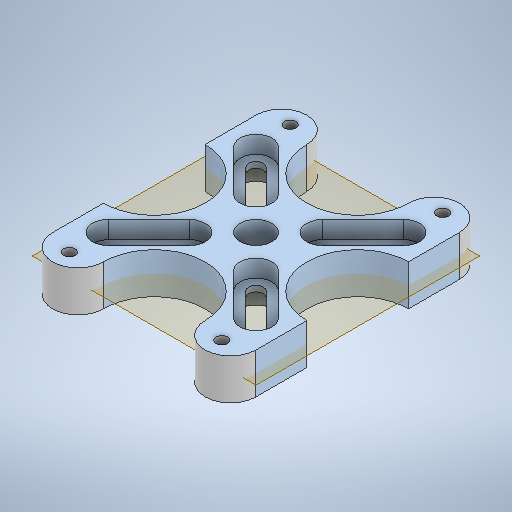
# Autodesk Inventor part: BaseSketchGrabberrev2.0
Saved by Autodesk Inventor 2025.1 (Build 291241000, 241)
## iProperties
Created: 2024-09-22
Part Number: BaseSketchGrabberrev2.0
Material: Generic
Document SubType Name: Modeling
Designer: m_kni
Density: 1 g/cm^3
Appearance: Default
Author: m_kni
Autodesk Inventor part; units mm, degrees
ref_plane "YZ Plane" through (0, 0, 0) normal (1, 0, 0) x (0, 1, 0)
ref_plane "XZ Plane" through (0, 0, 0) normal (0, 1, 0) x (-1, 0, 0)
ref_plane "XY Plane" through (0, 0, 0) normal (0, 0, 1) x (1, 0, 0)
sketch "Sketch1" plane through (0, 0, 0) normal (0, 1, 0) x (-1, 0, 0)
  line L0 (-12.7, 12.7) -> (12.7, 12.7)
  line L1 (12.7, 12.7) -> (12.7, -12.7)
  line L2 (12.7, -12.7) -> (-12.7, -12.7)
  line L3 (-12.7, -12.7) -> (-12.7, 12.7)
  line L4 (-12.7, 12.7) -> (12.7, -12.7) construction
  line L5 (12.7, 12.7) -> (-12.7, -12.7) construction
  line L6 (-11.4786, 11.4786) -> (11.4786, 11.4786)
  line L7 (11.4786, 11.4786) -> (11.4786, -11.4786)
  line L8 (11.4786, -11.4786) -> (-11.4786, -11.4786)
  line L9 (-11.4786, -11.4786) -> (-11.4786, 11.4786)
  line L10 (-11.4786, 11.4786) -> (11.4786, -11.4786) construction
  line L11 (11.4786, 11.4786) -> (-11.4786, -11.4786) construction
  line L12 (-25.4, -25.4) -> (25.4, -25.4)
  line L13 (25.4, -25.4) -> (25.4, 25.4)
  line L14 (25.4, 25.4) -> (-25.4, 25.4)
  line L15 (-25.4, 25.4) -> (-25.4, -25.4)
  line L16 (-25.4, -25.4) -> (25.4, 25.4) construction
  line L17 (25.4, -25.4) -> (-25.4, 25.4) construction
  circle A0 centre (0, 0) radius 5.5
  circle A1 centre (11.4786, 11.4786) radius 5.5
  circle A2 centre (11.4786, -11.4786) radius 5.5
  circle A3 centre (-11.4786, 11.4786) radius 5.5
  circle A4 centre (-11.4786, -11.4786) radius 5.5
  circle A5 centre (-25.4, 25.4) radius 5.5
  circle A6 centre (25.4, 25.4) radius 5.5
  circle A7 centre (25.4, -25.4) radius 5.5
  circle A8 centre (-25.4, -25.4) radius 5.5
  line L18 (7.5895, 15.3677) -> (21.5109, 29.2891)
  line L19 (29.2891, 21.5109) -> (15.3677, 7.5895)
  line L20 (15.3677, -7.5895) -> (29.2891, -21.5109)
  line L21 (-7.5895, -15.3677) -> (-21.5109, -29.2891)
  line L22 (-29.2891, 21.5109) -> (-15.3677, 7.5895)
  line L23 (7.5895, -15.3677) -> (21.5109, -29.2891)
  line L24 (-15.3677, -7.5895) -> (-29.2891, -21.5109)
  line L25 (-7.5895, 15.3677) -> (-21.5109, 29.2891)
  line L26 (-35, -35) -> (35, -35)
  line L27 (35, -35) -> (35, 35)
  line L28 (35, 35) -> (-35, 35)
  line L29 (-35, 35) -> (-35, -35)
  line L30 (-35, -35) -> (35, 35) construction
  line L31 (35, -35) -> (-35, 35) construction
  circle A9 centre (11.4786, 11.4786) radius 2.5
  circle A10 centre (25.4, 25.4) radius 2.5
  line L32 (27.1678, 23.6322) -> (13.2464, 9.7109)
  line L33 (23.6322, 27.1678) -> (9.7109, 13.2464)
  line L34 (0, 0) -> (0, 35)
  line L35 (35, 0) -> (0, 0)
  circle A11 centre (-11.4786, 11.4786) radius 2.5
  circle A12 centre (-25.4, 25.4) radius 2.5
  line L36 (-27.1678, 23.6322) -> (-13.2464, 9.7109)
  line L37 (-23.6322, 27.1678) -> (-9.7109, 13.2464)
  line L38 (25.4, 25.4) -> (-25.4, -25.4) construction
  circle A13 centre (11.4786, -11.4786) radius 2.5
  circle A14 centre (25.4, -25.4) radius 2.5
  line L39 (27.1678, -23.6322) -> (13.2464, -9.7109)
  line L40 (23.6322, -27.1678) -> (9.7109, -13.2464)
  line L41 (-27.1678, -23.6322) -> (-13.2464, -9.7109)
  circle A15 centre (-25.4, -25.4) radius 2.5
  line L42 (-23.6322, -27.1678) -> (-9.7109, -13.2464)
  circle A16 centre (-11.4786, -11.4786) radius 2.5
  dimension "d0" = 25.4
  dimension "d1" = 25.4
  dimension "d4" = 50.8
  dimension "d5" = 50.8
  dimension "d6" = 11
  dimension "d7" = 11
  dimension "d8" = 11
  dimension "d9" = 11
  dimension "d10" = 11
  dimension "d11" = 11
  dimension "d12" = 11
  dimension "d13" = 11
  dimension "d14" = 11
  dimension "d15" = 70
  dimension "d16" = 5
  dimension "d17" = 5
  constraints: 86 end point, 32 point on circle, 18 symmetric about line, 17 centre point, 13 tangent, 11 coincident, 10 midpoint, 8 parallel, 5 horizontal, 5 perpendicular, 3 point on line, 6 other
  measures "d0" distance of L1.end L2.end
  measures "d1" distance of L0.end L1.end
  measures "d4" distance of L14.end L13.end
  measures "d5" distance of L13.end L12.end
  measures "d6" diameter of A0
  measures "d7" diameter of A1
  measures "d8" diameter of A2
  measures "d9" diameter of A3
  measures "d10" diameter of A4
  measures "d11" diameter of A5
  measures "d12" diameter of A6
  measures "d13" diameter of A7
  measures "d14" diameter of A8
  measures "d15" distance of L28.end L27.end
  measures "d16" diameter of A9
  measures "d17" diameter of A10
extrude "Extrusion1" add sketch "Sketch1" along normal blind 14 contours A3 L25 L14 L34 L0 | L0 L34 L6 A3 | A3 L9 A4 L3 | L3 A4 L24 L15 L22 A3 | L34 L14 L18 A1 L0 | L0 A1 L6 L34 | L6 L34 A0 L35 L7 A2 L8 A4 L9 A3 | L6 A1 L7 L35 A0 L34 | L34 L28 L27 L35 L13 L19 A6 L18 L14 | L14 L25 A5 L22 L15 L24 A8 L21 L12 L23 A7 L20 L13 L35 L27 L26 L29 L28 L34 | L8 A2 L2 A4 | A1 L1 L35 L7 | L2 A2 L23 L12 L21 A4 | L35 L1 A2 L7 | A1 L19 L13 L35 L1 | L35 L13 L20 A2 L1
ref_plane "Work Plane1" through (0, 7, 0) normal (0, 1, 0) x (1, 0, 0)
sketch "Sketch3" plane through (0, 7, 0) normal (0, 1, 0) x (1, 0, 0)
  line L0 (-12.7, 12.7) -> (12.7, 12.7)
  line L1 (12.7, 12.7) -> (12.7, -12.7)
  line L2 (12.7, -12.7) -> (-12.7, -12.7)
  line L3 (-12.7, -12.7) -> (-12.7, 12.7)
  line L4 (-12.7, 12.7) -> (12.7, -12.7) construction
  line L5 (12.7, 12.7) -> (-12.7, -12.7) construction
  line L6 (-11.4786, 11.4786) -> (11.4786, 11.4786)
  line L7 (11.4786, 11.4786) -> (11.4786, -11.4786)
  line L8 (11.4786, -11.4786) -> (-11.4786, -11.4786)
  line L9 (-11.4786, -11.4786) -> (-11.4786, 11.4786)
  line L10 (-11.4786, 11.4786) -> (11.4786, -11.4786) construction
  line L11 (11.4786, 11.4786) -> (-11.4786, -11.4786) construction
  line L12 (-25.4, -25.4) -> (25.4, -25.4)
  line L13 (25.4, -25.4) -> (25.4, 25.4)
  line L14 (25.4, 25.4) -> (-25.4, 25.4)
  line L15 (-25.4, 25.4) -> (-25.4, -25.4)
  line L16 (-25.4, -25.4) -> (25.4, 25.4) construction
  line L17 (25.4, -25.4) -> (-25.4, 25.4) construction
  circle A0 centre (0, 0) radius 5.5
  circle A1 centre (11.4786, 11.4786) radius 5.5
  circle A2 centre (11.4786, -11.4786) radius 5.5
  circle A3 centre (-11.4786, 11.4786) radius 5.5
  circle A4 centre (-11.4786, -11.4786) radius 5.5
  circle A5 centre (-25.4, 25.4) radius 5.5
  circle A6 centre (25.4, 25.4) radius 5.5
  circle A7 centre (25.4, -25.4) radius 5.5
  circle A8 centre (-25.4, -25.4) radius 5.5
  line L18 (7.5895, 15.3677) -> (21.5109, 29.2891)
  line L19 (29.2891, 21.5109) -> (15.3677, 7.5895)
  line L20 (15.3677, -7.5895) -> (29.2891, -21.5109)
  line L21 (-7.5895, -15.3677) -> (-21.5109, -29.2891)
  line L22 (-29.2891, 21.5109) -> (-15.3677, 7.5895)
  line L23 (7.5895, -15.3677) -> (21.5109, -29.2891)
  line L24 (-15.719, -7.9759) -> (-29.6403, -21.8972)
  line L25 (-7.5895, 15.3677) -> (-21.5109, 29.2891)
  line L26 (-35, -35) -> (35, -35)
  line L27 (35, -35) -> (35, 35)
  line L28 (35, 35) -> (-35, 35)
  line L29 (-35, 35) -> (-35, -35)
  line L30 (-35, -35) -> (35, 35) construction
  line L31 (35, -35) -> (-35, 35) construction
  circle A9 centre (11.4786, 11.4786) radius 2.5
  circle A10 centre (25.4, 25.4) radius 2.5
  line L32 (27.1678, 23.6322) -> (13.2464, 9.7109)
  line L33 (23.58, 27.1139) -> (9.711, 13.2465)
  line L34 (0, 0) -> (0, 35)
  line L35 (35, 0) -> (0, 0)
  line L36 (-27.1678, 23.6322) -> (-13.2464, 9.7109)
  circle A11 centre (-25.4, 25.4) radius 2.5
  line L37 (-23.58, 27.1139) -> (-9.711, 13.2465)
  circle A12 centre (-11.4786, 11.4786) radius 2.5
  circle A13 centre (25.4, -25.4) radius 2.5
  line L38 (23.58, -27.1139) -> (9.711, -13.2465)
  line L39 (27.1678, -23.6322) -> (13.2464, -9.7109)
  circle A14 centre (11.4786, -11.4786) radius 2.5
  circle A15 centre (-11.4786, -11.4786) radius 2.5
  line L40 (-23.58, -27.1139) -> (-9.711, -13.2465)
  line L41 (-27.1678, -23.6322) -> (-13.2464, -9.7109)
  line L42 (25.4, 25.4) -> (-25.4, -25.4) construction
  circle A16 centre (-25.4, -25.4) radius 2.5
  point P0 (-23.7037, 20.1681)
  point P1 (-25.4, 19.9)
  point P2 (-25.4, 21.8645)
  point P3 (-21.8659, 25.4)
  point P4 (-19.9, 25.4)
  point P5 (-20.1684, 23.7028)
  dimension "d37" = 25.4
  dimension "d38" = 25.4
  dimension "d39" = 50.8
  dimension "d40" = 50.8
  dimension "d41" = 11
  dimension "d42" = 11
  dimension "d43" = 11
  dimension "d44" = 11
  dimension "d45" = 11
  dimension "d46" = 11
  dimension "d47" = 11
  dimension "d48" = 11
  dimension "d49" = 11
  dimension "d50" = 70
  dimension "d51" = 5
  dimension "d52" = 5
  constraints: 86 end point, 32 point on circle, 18 symmetric about line, 17 centre point, 14 tangent, 12 coincident, 10 midpoint, 8 parallel, 5 horizontal, 5 perpendicular, 3 point on line, 6 other
  measures "d37" distance of L1.end L2.end
  measures "d38" distance of L0.end L1.end
  measures "d39" distance of L14.end L13.end
  measures "d40" distance of L13.end L12.end
  measures "d41" diameter of A0
  measures "d42" diameter of A1
  measures "d43" diameter of A2
  measures "d44" diameter of A3
  measures "d45" diameter of A4
  measures "d46" diameter of A5
  measures "d47" diameter of A6
  measures "d48" diameter of A7
  measures "d49" diameter of A8
  measures "d50" distance of L28.end L27.end
  measures "d51" diameter of A9
  measures "d52" diameter of A10
extrude "Extrusion2" add sketch "Sketch3" along normal mid plane 2 contours A12 L37 A3 L0 | L0 A3 L6 A12 | A12 L9 A3 L3 | L3 A3 L36 A12 | L6 A3 L9 A12 | A3 L37 A5 L14 L25 | A4 L9 A15 L3 | L3 A15 L41 A4 | L22 L15 A5 L36 A3 | A1 L33 A9 L0 | L0 A9 L6 A1 | L14 A5 L25 | L37 L14 A5 | A4 L8 A15 L9 | A4 L41 A8 L15 L24 | L22 A5 L15 | A5 L15 L36 | L18 L14 A6 L33 A1 | L6 A9 L7 A1 | L18 A6 L14 | L14 L37 A11 L36 L15 A5 | A4 L2 A15 L8 | L15 A8 L24 | L7 A9 L1 A1 | A6 L13 L32 A10 L33 L14 | L14 L33 A6 | L2 A4 L40 A15 | A2 L7 A14 L8 | L8 A14 L2 A2 | A4 L21 L12 A8 L40 | L41 L15 A8 | L15 L41 A16 L40 L12 A8 L24 | A9 L32 A1 L1 | L32 A6 L13 L19 A1 | A2 L1 A14 L7 | L2 A14 L38 A2 | A8 L12 L40 | L32 L13 A6 | L19 L13 A6 | A2 L39 A14 L1 | A2 L38 A7 L12 L23 | L21 A8 L12 | L20 A7 L13 | L13 A7 L39 A2 L20 | L12 A7 L23 | A7 L12 L38 A13 L39 L13 | L13 L39 A7 | L38 L12 A7 picked at (-26.6909, 21.9384) picked at (26.6908, 21.9384) picked at (26.6909, -21.9384)
sketch "Sketch5" plane through (0, 14, 0) normal (0, 1, 0) x (1, 0, 0)
  line L0 (-35, 35) -> (-35, -35) projected
  circle A0 centre (-35, 0) radius 17.5
  line L1 (35, 35) -> (-35, 35) projected
  circle A1 centre (0, 35) radius 17.5
  line L2 (35, -35) -> (35, 35) projected
  circle A2 centre (35, 0) radius 17.5
  circle A3 centre (0, -35) radius 17.5
  point P0 (0, 0)
  point P1 (35, 17.5)
  point P2 (35, -17.5)
  point P3 (-17.5, 35)
  point P4 (17.5, 35)
  point P5 (-35, 17.5)
  point P6 (-35, -17.5)
  dimension "d79" = 35
  dimension "d80" = 35
  dimension "d81" = 35
  dimension "d82" = 35
  constraints: 4 centre point, 3 midpoint
  measures "d79" diameter of A0
  measures "d80" diameter of A1
  measures "d81" diameter of A2
  measures "d82" diameter of A3
extrude "Extrusion3" cut sketch "Sketch5" against normal blind 32.225 contours A0 L0 | A1 L1 | A2 L2 | A3 picked at (-31.363, 4.5607) picked at (-3.4832, 28.8033) picked at (32.2891, 5.1652)
sketch "Sketch7" plane through (0, 14, 0) normal (0, 1, 0) x (1, 0, 0)
  line L0 (-35, -35) -> (-17.5, -35) projected
  arc A0 (-35, -35) -> (-17.5, -35) centre (-26.25, -35) ccw
  point P0 (0, 0)
  constraints: 2 end point, 2 point on circle, 1 centre point, 1 midpoint
extrude "Extrusion4" add sketch "Sketch7" against normal blind 14
sketch "Sketch8" plane through (0, 14, 0) normal (0, 1, 0) x (1, 0, 0)
  arc A0 (-35, -35) -> (-17.5, -35) centre (-26.25, -35) ccw projected
  circle A1 centre (-26.25, -38) radius 2
  point P0 (0, 0)
  dimension "d89" = 4
  constraints: 1 centre point
  measures "d89" diameter of A1
extrude "Extrusion5" cut sketch "Sketch8" against normal blind 14
mirror "Mirror1" about plane through (0, 0, 0) normal (1, 0, 0) of "Extrusion5", "Extrusion4"
mirror "Mirror2" about plane through (0, 0, 0) normal (0, 0, 1) of "Extrusion4", "Extrusion5", "Mirror1"
body "Solid1"
